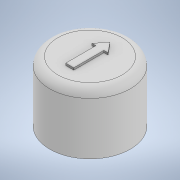
# Autodesk Inventor part: Device Direction Button
Saved by Autodesk Inventor 2021 (Build 250183000, 183)
## iProperties
Created: 2021-03-24
Part Number: Device Direction Button
Material: Generic
Document SubType Name: Modeling
Designer: eng1-127
Density: 1 g/cm^3
Appearance: Default
Author: eng1-127
Autodesk Inventor part; units mm, degrees
ref_plane "YZ Plane" through (0, 0, 0) normal (1, 0, 0) x (0, 1, 0)
ref_plane "XZ Plane" through (0, 0, 0) normal (0, 1, 0) x (-1, 0, 0)
ref_plane "XY Plane" through (0, 0, 0) normal (0, 0, 1) x (1, 0, 0)
sketch "Sketch1" plane through (0, 0, 0) normal (0, 1, 0) x (-1, 0, 0)
  circle A0 centre (0, 0) radius 10
  dimension "d0" = 20
  constraints: 1 centre point, 1 coincident
  measures "d0" diameter of A0
extrude "Extrusion1" add sketch "Sketch1" along normal blind 15
sketch "Sketch2" plane through (0, 0, 0) normal (0, -1, 0) x (1, 0, 0)
  circle A0 centre (0, 0) radius 7.5
  dimension "d3" = 15
  constraints: 1 centre point, 1 coincident
  measures "d3" diameter of A0
extrude "Extrusion2" cut sketch "Sketch2" against normal blind 5
fillet "Fillet1" radius 2 1 edges at (10, 15, 0)
sketch "Sketch3" plane through (0, 15, 0) normal (0, 1, 0) x (1, 0, 0)
  line L0 (-0.048, -4.9874) -> (-1.048, -4.9874)
  line L1 (-1.048, -4.9874) -> (-1.048, 2.5126)
  line L2 (-1.048, 2.5126) -> (-2.048, 2.5126)
  line L3 (-2.048, 2.5126) -> (-0.048, 5.0126)
  line L4 (-0.048, 5.0126) -> (-0.048, -4.9874)
  line L5 (-0.048, -4.9874) -> (0.952, -4.9874)
  line L6 (0.952, -4.9874) -> (0.952, 2.5126)
  line L7 (0.952, 2.5126) -> (1.952, 2.5126)
  line L8 (1.952, 2.5126) -> (-0.048, 5.0126)
  point P0 (0, 0)
  dimension "d7" = 1
  dimension "d8" = 7.5
  dimension "d9" = 10
  constraints: 18 end point, 3 symmetric about line, 2 perpendicular, 1 horizontal, 1 parallel
  measures "d7" distance of L0.start L0.end
  measures "d8" distance of L0.end L1.end
  measures "d9" distance of L3.end L0.start
extrude "Extrusion3" add sketch "Sketch3" along normal blind 0.5
body "Solid1"
